Autodesk Inventor part; units mm, degrees
(part 3 of 3)
  spline S382 degree 2 poles (128.7534, 1.3553) (128.7534, 1.4377) (128.7421, 1.5996) (128.7335, 1.6763) knots 0 0 0 1 2 2 2
  line L586 (128.7335, 1.6763) -> (127.3928, 0.6822)
  spline S383 degree 2 poles (127.3928, 0.6822) (127.4269, 0.5543) (127.5405, 0.3413) (127.6968, 0.1879) (127.8984, 0.1027) (128.0291, 0.1027) knots 0 0 0 1 2 3 4 4 4
  spline S384 degree 2 poles (128.0291, 0.1027) (128.1938, 0.1027) (128.4609, 0.2618) (128.6512, 0.5799) (128.7534, 1.0486) (128.7534, 1.3553) knots 0 0 0 1 2 3 4 4 4
  spline S385 degree 2 poles (127.3019, 1.3838) (127.3019, 1.3099) (127.3048, 1.1594) (127.3104, 1.0883) knots 0 0 0 1 2 2 2
  line L587 (127.3104, 1.0883) -> (128.654, 2.0797)
  spline S386 degree 2 poles (128.654, 2.0797) (128.6171, 2.2047) (128.5063, 2.4092) (128.3501, 2.5569) (128.1512, 2.6393) (128.0291, 2.6393) knots 0 0 0 1 2 3 4 4 4
  spline S387 degree 2 poles (128.0291, 2.6393) (127.8615, 2.6393) (127.5945, 2.4802) (127.4042, 2.1621) (127.3019, 1.6934) (127.3019, 1.3838) knots 0 0 0 1 2 3 4 4 4
  line L588 (131.5229, -0.2154) -> (131.5229, 1.5343)
  spline S388 degree 2 poles (131.5229, 1.5343) (131.5229, 1.6479) (131.5059, 1.7928) (131.4718, 1.878) (131.4207, 1.9121) (131.3809, 1.9121) knots 0 0 0 1 2 3 4 4 4
  spline S389 degree 2 poles (131.3809, 1.9121) (131.3354, 1.9121) (131.2587, 1.8553) (131.1707, 1.7218) (131.0656, 1.5059) (130.9917, 1.3497) knots 0 0 0 1 2 3 4 4 4
  line L589 (130.9917, 1.3497) -> (130.9917, -0.2154)
  line L590 (130.9917, -0.2154) -> (130.5685, -0.2154)
  line L591 (130.5685, -0.2154) -> (130.5685, 1.4889)
  spline S390 degree 2 poles (130.5685, 1.4889) (130.5685, 1.6224) (130.5515, 1.7871) (130.5174, 1.878) (130.4634, 1.9121) (130.4236, 1.9121) knots 0 0 0 1 2 3 4 4 4
  spline S391 degree 2 poles (130.4236, 1.9121) (130.3839, 1.9121) (130.31, 1.8638) (130.222, 1.7388) (130.1112, 1.5201) (130.0373, 1.3497) knots 0 0 0 1 2 3 4 4 4
  line L592 (130.0373, 1.3497) -> (130.0373, -0.2154)
  line L593 (130.0373, -0.2154) -> (129.6141, -0.2154)
  line L594 (129.6141, -0.2154) -> (129.6141, 2.2189)
  line L595 (129.6141, 2.2189) -> (129.9663, 2.2189)
  line L596 (129.9663, 2.2189) -> (129.9862, 1.7559)
  spline S392 degree 2 poles (129.9862, 1.7559) (130.0515, 1.895) (130.1708, 2.0882) (130.2958, 2.2075) (130.4407, 2.2643) (130.5259, 2.2643) knots 0 0 0 1 2 3 4 4 4
  spline S393 degree 2 poles (130.5259, 2.2643) (130.7247, 2.2643) (130.9292, 2.0058) (130.9292, 1.736) knots 0 0 0 1 2 2 2
  spline S394 degree 2 poles (130.9292, 1.736) (130.9861, 1.8638) (131.0997, 2.0598) (131.2275, 2.1933) (131.3837, 2.2643) (131.486, 2.2643) knots 0 0 0 1 2 3 4 4 4
  spline S395 degree 2 poles (131.486, 2.2643) (131.9461, 2.2643) (131.9461, 1.557) knots 0 0 0 1 1 1
  line L597 (131.9461, 1.557) -> (131.9461, -0.2154)
  line L598 (131.9461, -0.2154) -> (131.5229, -0.2154)
  line L599 (134.8378, -0.2154) -> (134.3663, -0.2154)
  line L600 (134.3663, -0.2154) -> (134.1475, 0.4748)
  line L601 (134.1475, 0.4748) -> (132.821, 0.4748)
  line L602 (132.821, 0.4748) -> (132.5995, -0.2154)
  line L603 (132.5995, -0.2154) -> (132.1535, -0.2154)
  line L604 (132.1535, -0.2154) -> (133.2045, 2.9546)
  line L605 (133.2045, 2.9546) -> (133.7982, 2.9546)
  line L606 (133.7982, 2.9546) -> (134.8378, -0.2154)
  line L607 (134.0226, 0.8611) -> (133.4857, 2.5597)
  line L608 (133.4857, 2.5597) -> (132.9432, 0.8611)
  line L609 (132.9432, 0.8611) -> (134.0226, 0.8611)
  line L610 (114.9596, -5.248) -> (113.2868, -5.248)
  line L611 (113.2868, -5.248) -> (113.2868, -4.9453)
  line L612 (113.2868, -4.9453) -> (113.9423, -4.2921)
  spline S396 degree 2 poles (113.9423, -4.2921) (114.1039, -4.1328) (114.3064, -3.8984) (114.4179, -3.7049) (114.4566, -3.5342) (114.4566, -3.4363) knots 0 0 0 1 2 3 4 4 4
  spline S397 degree 2 poles (114.4566, -3.4363) (114.4566, -3.343) (114.4066, -3.1746) (114.3019, -3.0449) (114.1334, -2.972) (114.0174, -2.972) knots 0 0 0 1 2 3 4 4 4
  spline S398 degree 2 poles (114.0174, -2.972) (113.8558, -2.972) (113.5918, -3.1154) (113.4825, -3.2315) knots 0 0 0 1 2 2 2
  line L613 (113.4825, -3.2315) -> (113.2959, -3.0062)
  spline S399 degree 2 poles (113.2959, -3.0062) (113.4393, -2.856) (113.8148, -2.6716) (114.0629, -2.6716) knots 0 0 0 1 2 2 2
  spline S400 degree 2 poles (114.0629, -2.6716) (114.2313, -2.6716) (114.5113, -2.7718) (114.7115, -2.9629) (114.8231, -3.2383) (114.8231, -3.4113) knots 0 0 0 1 2 3 4 4 4
  spline S401 degree 2 poles (114.8231, -3.4113) (114.8231, -3.5592) (114.7457, -3.8073) (114.5886, -4.0531) (114.3497, -4.3171) (114.1858, -4.4765) knots 0 0 0 1 2 3 4 4 4
  line L614 (114.1858, -4.4765) -> (113.726, -4.9248)
  line L615 (113.726, -4.9248) -> (114.9596, -4.9248)
  line L616 (114.9596, -4.9248) -> (114.9596, -5.248)
  line L617 (117.2766, -4.6859) -> (116.8419, -4.6859)
  line L618 (116.8419, -4.6859) -> (116.8419, -5.248)
  line L619 (116.8419, -5.248) -> (116.4959, -5.248)
  line L620 (116.4959, -5.248) -> (116.4959, -4.6859)
  line L621 (116.4959, -4.6859) -> (115.2737, -4.6859)
  line L622 (115.2737, -4.6859) -> (115.2737, -4.3877)
  line L623 (115.2737, -4.3877) -> (116.3571, -2.708)
  line L624 (116.3571, -2.708) -> (116.8419, -2.708)
  line L625 (116.8419, -2.708) -> (116.8419, -4.3877)
  line L626 (116.8419, -4.3877) -> (117.2766, -4.3877)
  line L627 (117.2766, -4.3877) -> (117.2766, -4.6859)
  line L628 (116.4959, -3.0335) -> (115.6128, -4.3877)
  line L629 (115.6128, -4.3877) -> (116.4959, -4.3877)
  line L630 (116.4959, -4.3877) -> (116.4959, -3.0335)
  line L631 (117.511, -3.2975) -> (117.8956, -3.2975)
  line L632 (117.8956, -3.2975) -> (118.3713, -4.588)
  line L633 (118.3713, -4.588) -> (118.476, -4.9044)
  line L634 (118.476, -4.9044) -> (118.5807, -4.5812)
  line L635 (118.5807, -4.5812) -> (119.0541, -3.2975)
  line L636 (119.0541, -3.2975) -> (119.4274, -3.2975)
  line L637 (119.4274, -3.2975) -> (118.6604, -5.248)
  line L638 (118.6604, -5.248) -> (118.2735, -5.248)
  line L639 (118.2735, -5.248) -> (117.511, -3.2975)
  spline S402 degree 2 poles (121.6146, -3.9507) (121.6146, -4.1328) (121.5577, -4.4674) (121.4348, -4.7541) (121.2368, -4.9886) (120.9477, -5.157) (120.5677, -5.248) (120.3241, -5.248) knots 0 0 0 1 2 3 4 5 6 6 6
  line L640 (120.3241, -5.248) -> (119.7802, -5.248)
  line L641 (119.7802, -5.248) -> (119.7802, -2.708)
  line L642 (119.7802, -2.708) -> (120.4356, -2.708)
  spline S403 degree 2 poles (120.4356, -2.708) (121.0297, -2.708) (121.6146, -3.3203) (121.6146, -3.9507) knots 0 0 0 1 2 2 2
  spline S404 degree 2 poles (121.2504, -3.9735) (121.2504, -3.7049) (121.1503, -3.3316) (120.9432, -3.1018) (120.6337, -2.9994) (120.4243, -2.9994) knots 0 0 0 1 2 3 4 4 4
  line L643 (120.4243, -2.9994) -> (120.1261, -2.9994)
  line L644 (120.1261, -2.9994) -> (120.1261, -4.9476)
  line L645 (120.1261, -4.9476) -> (120.3833, -4.9476)
  spline S405 degree 2 poles (120.3833, -4.9476) (121.2504, -4.9476) (121.2504, -3.9735) knots 0 0 0 1 1 1
  spline S406 degree 2 poles (123.6926, -5.1524) (123.3876, -5.2799) (123.053, -5.2799) knots 0 0 0 1 1 1
  spline S407 degree 2 poles (123.053, -5.2799) (122.5159, -5.2799) (121.9378, -4.6358) (121.9378, -4.0053) knots 0 0 0 1 2 2 2
  spline S408 degree 2 poles (121.9378, -4.0053) (121.9378, -3.7004) (122.0971, -3.2065) (122.393, -2.8628) (122.8118, -2.6762) (123.0735, -2.6762) knots 0 0 0 1 2 3 4 4 4
  spline S409 degree 2 poles (123.0735, -2.6762) (123.2488, -2.6762) (123.5537, -2.7376) (123.6926, -2.7991) knots 0 0 0 1 2 2 2
  line L646 (123.6926, -2.7991) -> (123.6926, -3.1382)
  spline S410 degree 2 poles (123.6926, -3.1382) (123.5537, -3.0631) (123.2579, -2.9834) (123.0849, -2.9834) knots 0 0 0 1 2 2 2
  spline S411 degree 2 poles (123.0849, -2.9834) (122.9051, -2.9834) (122.616, -3.1177) (122.4135, -3.3726) (122.3042, -3.739) (122.3042, -3.9757) knots 0 0 0 1 2 3 4 4 4
  spline S412 degree 2 poles (122.3042, -3.9757) (122.3042, -4.4696) (122.7048, -4.9704) (123.0917, -4.9704) knots 0 0 0 1 2 2 2
  spline S413 degree 2 poles (123.0917, -4.9704) (123.2556, -4.9704) (123.5537, -4.8952) (123.6926, -4.827) knots 0 0 0 1 2 2 2
  line L647 (123.6926, -4.827) -> (123.6926, -5.1524)
  spline S414 degree 2 poles (127.6141, -6.0651) (126.7196, -5.2344) (126.7196, -4.2284) knots 0 0 0 1 1 1
  spline S415 degree 2 poles (126.7196, -4.2284) (126.7196, -3.994) (126.8152, -3.5251) (127.0269, -3.054) (127.3751, -2.5851) (127.6232, -2.353) knots 0 0 0 1 2 3 4 4 4
  line L648 (127.6232, -2.353) -> (127.8189, -2.5533)
  spline S416 degree 2 poles (127.8189, -2.5533) (127.0656, -3.2975) (127.0656, -4.2033) knots 0 0 0 1 1 1
  spline S417 degree 2 poles (127.0656, -4.2033) (127.0656, -4.6563) (127.4457, -5.487) (127.8189, -5.858) knots 0 0 0 1 2 2 2
  line L649 (127.8189, -5.858) -> (127.6141, -6.0651)
  line L650 (130.4204, -5.248) -> (130.0813, -5.248)
  line L651 (130.0813, -5.248) -> (130.0312, -3.6617)
  line L652 (130.0312, -3.6617) -> (130.0107, -3.0563)
  line L653 (130.0107, -3.0563) -> (129.8924, -3.409)
  line L654 (129.8924, -3.409) -> (129.5168, -4.4196)
  line L655 (129.5168, -4.4196) -> (129.2778, -4.4196)
  line L656 (129.2778, -4.4196) -> (128.9205, -3.4477)
  line L657 (128.9205, -3.4477) -> (128.8044, -3.0563)
  line L658 (128.8044, -3.0563) -> (128.7953, -3.689)
  line L659 (128.7953, -3.689) -> (128.7498, -5.248)
  line L660 (128.7498, -5.248) -> (128.4244, -5.248)
  line L661 (128.4244, -5.248) -> (128.5495, -2.708)
  line L662 (128.5495, -2.708) -> (128.9592, -2.708)
  line L663 (128.9592, -2.708) -> (129.3006, -3.6639)
  line L664 (129.3006, -3.6639) -> (129.4099, -3.9871)
  line L665 (129.4099, -3.9871) -> (129.5168, -3.6639)
  line L666 (129.5168, -3.6639) -> (129.8764, -2.708)
  line L667 (129.8764, -2.708) -> (130.2975, -2.708)
  line L668 (130.2975, -2.708) -> (130.4204, -5.248)
  line L669 (132.0819, -5.248) -> (132.075, -4.9863)
  spline S418 degree 2 poles (132.075, -4.9863) (131.9157, -5.1433) (131.5857, -5.2822) (131.4059, -5.2822) knots 0 0 0 1 2 2 2
  spline S419 degree 2 poles (131.4059, -5.2822) (131.2375, -5.2822) (131.0008, -5.1957) (130.8483, -5.0477) (130.7754, -4.8452) (130.7754, -4.7268) knots 0 0 0 1 2 3 4 4 4
  spline S420 degree 2 poles (130.7754, -4.7268) (130.7754, -4.4332) (131.2124, -4.1009) (131.6403, -4.1009) knots 0 0 0 1 2 2 2
  line L670 (131.6403, -4.1009) -> (132.0454, -4.1009)
  line L671 (132.0454, -4.1009) -> (132.0454, -3.9302)
  spline S421 degree 2 poles (132.0454, -3.9302) (132.0454, -3.7573) (131.8247, -3.5479) (131.5971, -3.5479) knots 0 0 0 1 2 2 2
  spline S422 degree 2 poles (131.5971, -3.5479) (131.4309, -3.5479) (131.11, -3.6207) (130.9393, -3.689) knots 0 0 0 1 2 2 2
  line L672 (130.9393, -3.689) -> (130.9393, -3.384)
  spline S423 degree 2 poles (130.9393, -3.384) (131.003, -3.3612) (131.1601, -3.3157) (131.3353, -3.2816) (131.5265, -3.2611) (131.6221, -3.2611) knots 0 0 0 1 2 3 4 4 4
  spline S424 degree 2 poles (131.6221, -3.2611) (131.7996, -3.2611) (132.0841, -3.3385) (132.2799, -3.4978) (132.3846, -3.739) (132.3846, -3.9029) knots 0 0 0 1 2 3 4 4 4
  line L673 (132.3846, -3.9029) -> (132.3846, -5.248)
  line L674 (132.3846, -5.248) -> (132.0819, -5.248)
  line L675 (132.0454, -4.3604) -> (131.6153, -4.3604)
  spline S425 degree 2 poles (131.6153, -4.3604) (131.4878, -4.3604) (131.3058, -4.4105) (131.1897, -4.5038) (131.1328, -4.6335) (131.1328, -4.7154) knots 0 0 0 1 2 3 4 4 4
  spline S426 degree 2 poles (131.1328, -4.7154) (131.1328, -4.7723) (131.1669, -4.8748) (131.2466, -4.9544) (131.3695, -4.9999) (131.4605, -4.9999) knots 0 0 0 1 2 3 4 4 4
  spline S427 degree 2 poles (131.4605, -4.9999) (131.5766, -4.9999) (131.877, -4.8588) (132.0454, -4.7063) knots 0 0 0 1 2 2 2
  line L676 (132.0454, -4.7063) -> (132.0454, -4.3604)
  line L677 (134.7766, -5.248) -> (134.3283, -5.248)
  line L678 (134.3283, -5.248) -> (133.8002, -4.5061)
  line L679 (133.8002, -4.5061) -> (133.279, -5.248)
  line L680 (133.279, -5.248) -> (132.842, -5.248)
  line L681 (132.842, -5.248) -> (133.5999, -4.2694)
  line L682 (133.5999, -4.2694) -> (132.8762, -3.2975)
  line L683 (132.8762, -3.2975) -> (133.3086, -3.2975)
  line L684 (133.3086, -3.2975) -> (133.823, -4.0486)
  line L685 (133.823, -4.0486) -> (134.326, -3.2975)
  line L686 (134.326, -3.2975) -> (134.7448, -3.2975)
  line L687 (134.7448, -3.2975) -> (134.0119, -4.2762)
  line L688 (134.0119, -4.2762) -> (134.7766, -5.248)
  spline S428 degree 2 poles (135.6051, -2.353) (136.5018, -3.1837) (136.5018, -4.2011) knots 0 0 0 1 1 1
  spline S429 degree 2 poles (136.5018, -4.2011) (136.5018, -4.4105) (136.4153, -4.8611) (136.2105, -5.3345) (135.8623, -5.8193) (135.596, -6.0651) knots 0 0 0 1 2 3 4 4 4
  line L689 (135.596, -6.0651) -> (135.4003, -5.8648)
  spline S430 degree 2 poles (135.4003, -5.8648) (135.7803, -5.4893) (136.1536, -4.6722) (136.1536, -4.2261) knots 0 0 0 1 2 2 2
  spline S431 degree 2 poles (136.1536, -4.2261) (136.1536, -3.2998) (135.4003, -2.5601) knots 0 0 0 1 1 1
  line L690 (135.4003, -2.5601) -> (135.6051, -2.353)
  line L691 (120.7098, -38.17) -> (120.2383, -38.17)
  line L692 (120.2383, -38.17) -> (120.0196, -37.4798)
  line L693 (120.0196, -37.4798) -> (118.6931, -37.4798)
  line L694 (118.6931, -37.4798) -> (118.4715, -38.17)
  line L695 (118.4715, -38.17) -> (118.0256, -38.17)
  line L696 (118.0256, -38.17) -> (119.0766, -35)
  line L697 (119.0766, -35) -> (119.6702, -35)
  line L698 (119.6702, -35) -> (120.7098, -38.17)
  line L699 (119.8946, -37.0934) -> (119.3578, -35.3948)
  line L700 (119.3578, -35.3948) -> (118.8152, -37.0934)
  line L701 (118.8152, -37.0934) -> (119.8946, -37.0934)
  line L702 (121.8801, -35.3636) -> (121.1501, -35.3636)
  line L703 (121.1501, -35.3636) -> (121.1501, -35)
  line L704 (121.1501, -35) -> (123.0476, -35)
  line L705 (123.0476, -35) -> (123.0476, -35.3636)
  line L706 (123.0476, -35.3636) -> (122.3176, -35.3636)
  line L707 (122.3176, -35.3636) -> (122.3176, -37.8007)
  line L708 (122.3176, -37.8007) -> (123.0476, -37.8007)
  line L709 (123.0476, -37.8007) -> (123.0476, -38.17)
  line L710 (123.0476, -38.17) -> (121.1501, -38.17)
  line L711 (121.1501, -38.17) -> (121.1501, -37.8007)
  line L712 (121.1501, -37.8007) -> (121.8801, -37.8007)
  line L713 (121.8801, -37.8007) -> (121.8801, -35.3636)
  line L714 (128.8024, -37.4684) -> (128.2599, -37.4684)
  line L715 (128.2599, -37.4684) -> (128.2599, -38.17)
  line L716 (128.2599, -38.17) -> (127.8281, -38.17)
  line L717 (127.8281, -38.17) -> (127.8281, -37.4684)
  line L718 (127.8281, -37.4684) -> (126.3028, -37.4684)
  line L719 (126.3028, -37.4684) -> (126.3028, -37.0963)
  line L720 (126.3028, -37.0963) -> (127.6549, -35)
  line L721 (127.6549, -35) -> (128.2599, -35)
  line L722 (128.2599, -35) -> (128.2599, -37.0963)
  line L723 (128.2599, -37.0963) -> (128.8024, -37.0963)
  line L724 (128.8024, -37.0963) -> (128.8024, -37.4684)
  line L725 (127.8281, -35.4062) -> (126.726, -37.0963)
  line L726 (126.726, -37.0963) -> (127.8281, -37.0963)
  line L727 (127.8281, -37.0963) -> (127.8281, -35.4062)
  line L728 (75.7098, -38.2154) -> (75.2383, -38.2154)
  line L729 (75.2383, -38.2154) -> (75.0196, -37.5252)
  line L730 (75.0196, -37.5252) -> (73.6931, -37.5252)
  line L731 (73.6931, -37.5252) -> (73.4715, -38.2154)
  line L732 (73.4715, -38.2154) -> (73.0256, -38.2154)
  line L733 (73.0256, -38.2154) -> (74.0766, -35.0454)
  line L734 (74.0766, -35.0454) -> (74.6702, -35.0454)
  line L735 (74.6702, -35.0454) -> (75.7098, -38.2154)
  line L736 (74.8946, -37.1389) -> (74.3578, -35.4403)
  line L737 (74.3578, -35.4403) -> (73.8152, -37.1389)
  line L738 (73.8152, -37.1389) -> (74.8946, -37.1389)
  line L739 (76.8801, -35.409) -> (76.1501, -35.409)
  line L740 (76.1501, -35.409) -> (76.1501, -35.0454)
  line L741 (76.1501, -35.0454) -> (78.0476, -35.0454)
  line L742 (78.0476, -35.0454) -> (78.0476, -35.409)
  line L743 (78.0476, -35.409) -> (77.3176, -35.409)
  line L744 (77.3176, -35.409) -> (77.3176, -37.8462)
  line L745 (77.3176, -37.8462) -> (78.0476, -37.8462)
  line L746 (78.0476, -37.8462) -> (78.0476, -38.2154)
  line L747 (78.0476, -38.2154) -> (76.1501, -38.2154)
  line L748 (76.1501, -38.2154) -> (76.1501, -37.8462)
  line L749 (76.1501, -37.8462) -> (76.8801, -37.8462)
  line L750 (76.8801, -37.8462) -> (76.8801, -35.409)
  line L751 (83.6434, -38.2154) -> (81.5556, -38.2154)
  line L752 (81.5556, -38.2154) -> (81.5556, -37.8377)
  line L753 (81.5556, -37.8377) -> (82.3737, -37.0224)
  spline S432 degree 2 poles (82.3737, -37.0224) (82.5753, -36.8236) (82.8281, -36.531) (82.9673, -36.2896) (83.0156, -36.0766) (83.0156, -35.9544) knots 0 0 0 1 2 3 4 4 4
  spline S433 degree 2 poles (83.0156, -35.9544) (83.0156, -35.8379) (82.9531, -35.6278) (82.8225, -35.4658) (82.6123, -35.3749) (82.4674, -35.3749) knots 0 0 0 1 2 3 4 4 4
  spline S434 degree 2 poles (82.4674, -35.3749) (82.2657, -35.3749) (81.9362, -35.5539) (81.7999, -35.6988) knots 0 0 0 1 2 2 2
  line L754 (81.7999, -35.6988) -> (81.567, -35.4176)
  spline S435 degree 2 poles (81.567, -35.4176) (81.7459, -35.2301) (82.2146, -35) (82.5242, -35) knots 0 0 0 1 2 2 2
  spline S436 degree 2 poles (82.5242, -35) (82.7344, -35) (83.0838, -35.125) (83.3337, -35.3636) (83.4729, -35.7073) (83.4729, -35.9232) knots 0 0 0 1 2 3 4 4 4
  spline S437 degree 2 poles (83.4729, -35.9232) (83.4729, -36.1078) (83.3764, -36.4174) (83.1804, -36.7242) (82.8821, -37.0537) (82.6776, -37.2525) knots 0 0 0 1 2 3 4 4 4
  line L755 (82.6776, -37.2525) -> (82.1038, -37.8121)
  line L756 (82.1038, -37.8121) -> (83.6434, -37.8121)
  line L757 (83.6434, -37.8121) -> (83.6434, -38.2154)
  point P0 (0, 0)
  dimension "d66" = 10
  dimension "d67" = 10
  dimension "d68" = 5
  dimension "d69" = 5
  dimension "d70" = 10
  dimension "d71" = 6
  dimension "d72" = 6
  dimension "d73" = 10
  dimension "d74" = 27
  dimension "d75" = 11
  dimension "d76" = 11
  dimension "d77" = 11
  dimension "d79" = 11
  dimension "d80" = 10
  dimension "d81" = 10
  dimension "d82" = 23
  dimension "d83" = 23
  dimension "d84" = 4
  constraints: 6 horizontal alignment, 4 vertical alignment, 2 horizontal, 28 other
  measures "d66" distance from line of L13 A0.centre
  measures "d67" distance from line of L21 A1.centre
  measures "d68" distance from line of L12 A0.centre
  measures "d69" distance from line of A2.centre L16
  measures "d70" distance from line of L41 A3.centre
  measures "d71" distance from line of A3.centre L40
  measures "d72" distance from line of L48 A4.centre
  measures "d73" distance from line of A5.centre L45
  measures "d74" distance from line of A3.centre L29
  measures "d75" distance from line of A3.centre L28
  measures "d76" distance from line of A4.centre L32
  measures "d77" distance from line of A4.centre L36
  measures "d79" distance between parallel lines of L56 L4
  measures "d80" distance between parallel lines of L57 L7
  measures "d81" distance between parallel lines of L58 L5
  measures "d82" distance from line of A6.centre L8
  measures "d83" distance from line of L10 A6.centre
  measures "d84" distance between parallel lines of L59 L0
extrude "Extrusion4" cut sketch "Sketch5" against normal blind 10 contours L60 L61 L62 L63 L64 L65 | L66 S0 S1 S2 L67 L68 S3 S4 L69 S5 S6 L70 L71 | S10 S11 L74 L75 L76 L77 S12 S13 | L79 L80 L81 L82 L83 L84 L85 L86 L87 | L88 L89 L90 L91 L92 L93 L94 L95 L96 L97 L98 L99 | L100 L101 L102 L103 L104 L105 L106 L107 L108 L109 L110 L111 | L112 L113 L114 L115 L116 L117 L118 L119 L120 L121 L122 L123 L124 L125 L126 L127 L128 L129 L130 | L131 L132 L133 L134 L135 L136 L137 L138 | L139 L140 S18 S19 L141 S20 S21 L142 L143 L144 | L145 S22 S23 S24 L146 L147 S25 S26 L148 S27 S28 L149 L150 | L153 L154 L155 L156 L157 L158 L159 L160 L161 L162 | S32 S33 S34 S35 | L163 L164 S36 S37 L165 L166 L167 S38 S39 L168 L169 L170 | L171 L172 L173 L174 L175 L176 L177 L178 L179 L180 | S40 S41 S42 S43 | L181 L182 S44 S45 L183 L184 L185 S46 S47 L186 L187 L188 | S48 S49 S50 S51 S52 L189 S53 S54 S55 S56 S57 S58 S59 S60 S61 L190 L191 L192 | L194 L195 S70 L196 L197 L198 L199 L200 S71 S72 S73 L201 | L205 L206 L207 L208 L209 L210 L211 L212 L213 L214 | S76 S77 S78 S79 | S80 S81 S82 S83 S84 L215 S85 S86 S87 S88 S89 S90 S91 S92 S93 L216 L217 L218 | L220 L221 L222 L223 L224 L225 L226 L227 | L231 S102 S103 L232 L233 L234 S104 S105 L235 L236 L237 L238 L239 S106 S107 S108 S109 L240 L241 | S110 S111 L242 L243 L244 L245 L246 S112 S113 | L248 S118 S119 L249 L250 L251 S120 S121 L252 L253 L254 L255 L256 S122 S123 S124 S125 L257 L258 | S126 L259 S127 S128 L260 S129 S130 S131 S132 | S135 S136 L262 L263 L264 L265 L266 L267 L268 L269 L270 L271 L272 S137 S138 L273 | S139 L274 S140 S141 L275 S142 S143 S144 S145 | L277 L278 S148 S149 L279 S150 S151 L280 L281 L282 | S152 S153 S154 S155 | L285 L286 L287 L288 | L289 L290 L291 S162 S163 S164 L292 S165 S166 S167 L293 L294 L295 | S168 S169 S170 S171 | L298 S178 S179 L299 L300 L301 S180 S181 L302 L303 L304 L305 L306 S182 S183 S184 S185 L307 L308 | L309 L310 L311 L312 L313 L314 L315 L316 | L320 L321 L322 L323 L324 L325 L326 L327 L328 | S186 S187 S188 S189 | L329 L330 L331 L332 L333 L334 L335 L336 L337 L338 | S194 S195 L339 L340 L341 L342 L343 L344 L345 L346 L347 L348 L349 S196 S197 L350 | L351 S198 S199 L352 L353 L354 S200 S201 L355 L356 L357 L358 L359 S202 S203 S204 S205 L360 L361 | S206 L362 S207 S208 L363 S209 S210 S211 S212 | S215 S216 L365 L366 L367 L368 L369 L370 L371 L372 L373 L374 L375 S217 S218 L376 | S219 L377 S220 S221 L378 S222 S223 S224 S225 | L380 L381 S228 S229 L382 S230 S231 L383 L384 L385 | S232 S233 S234 S235 | L388 L389 L390 L391 | L392 L393 L394 L395 L396 L397 L398 L399 L400 L401 L402 | S242 S243 S244 S245 | L405 L406 L407 L408 L409 L410 L411 L412 L413 | S252 L414 L415 L416 S253 | S256 S257 S258 S259 | S264 S265 L420 S266 S267 S268 L421 L422 L423 S269 S270 S271 L424 S272 S273 S274 S275 | S276 L425 L426 L427 S277 | S280 S281 S282 S283 | L431 L432 L433 L434 L435 L436 L437 L438 L439 L440 L441 | S288 L442 L443 L444 S289 | S292 S293 S294 S295 | L448 L449 L450 S300 S301 S302 L451 S303 S304 S305 L452 L453 L454 | S306 L455 L456 L457 S307 | S310 S311 S312 S313 | L461 L462 L463 L464 L465 L466 L467 L468 L469 L470 L471 | L475 L476 L477 L478 L479 L480 L481 L482 | L486 L487 L488 L489 L490 L491 L492 L493 L494 L495 L496 L497 | L498 L499 L500 L501 L502 L503 L504 L505 L506 L507 L508 | S318 S319 S320 S321 | L511 L512 L513 L514 | L515 L516 L517 L518 L519 L520 L521 L522 L523 L524 L525 | S328 S329 S330 S331 | L528 L529 L530 L531 L532 L533 L534 L535 L536 | S338 L537 L538 L539 S339 | S342 S343 S344 S345 L543 S346 S347 S348 S349 L544 | L545 L546 L547 L548 L549 L550 L551 L552 | L556 L557 L558 L559 L560 L561 L562 L563 L564 L565 L566 L567 | S350 S351 L568 S352 S353 S354 L569 L570 L571 S355 S356 S357 L572 S358 S359 S360 S361 | S362 S363 S364 S365 | L575 L576 L577 L578 | L579 L580 L581 S372 S373 S374 L582 S375 S376 S377 L583 L584 L585 | S378 S379 S380 S381 | L588 S388 S389 L589 L590 L591 S390 S391 L592 L593 L594 L595 L596 S392 S393 S394 S395 L597 L598 | L599 L600 L601 L602 L603 L604 L605 L606 | L610 L611 L612 S396 S397 S398 L613 S399 S400 S401 L614 L615 L616 | L617 L618 L619 L620 L621 L622 L623 L624 L625 L626 L627 | L631 L632 L633 L634 L635 L636 L637 L638 L639 | S402 L640 L641 L642 S403 | S406 S407 S408 S409 L646 S410 S411 S412 S413 L647 | S414 S415 L648 S416 S417 L649 | L650 L651 L652 L653 L654 L655 L656 L657 L658 L659 L660 L661 L662 L663 L664 L665 L666 L667 L668 | L669 S418 S419 S420 L670 L671 S421 S422 L672 S423 S424 L673 L674 | L677 L678 L679 L680 L681 L682 L683 L684 L685 L686 L687 L688 | S428 S429 L689 S430 S431 L690 | L691 L692 L693 L694 L695 L696 L697 L698 | L702 L703 L704 L705 L706 L707 L708 L709 L710 L711 L712 L713 | L714 L715 L716 L717 L718 L719 L720 L721 L722 L723 L724 | L728 L729 L730 L731 L732 L733 L734 L735 | L739 L740 L741 L742 L743 L744 L745 L746 L747 L748 L749 L750 | L751 L752 L753 S432 S433 S434 L754 S435 S436 S437 L755 L756 L757
sketch "Sketch6" plane through (0, 5, 0) normal (0, 1, 0) x (1, 0, 0)
  line L0 (79, 30) -> (79, -25) construction
  line L1 (63, 30) -> (63, -25)
  line L2 (95, -25) -> (95, 30)
  arc A0 (95, 30) -> (63, 30) centre (79, 30) ccw
  arc A1 (63, -25) -> (95, -25) centre (79, -25) ccw
  line L3 (124, 30) -> (124, -25) construction
  line L4 (108, 30) -> (108, -25)
  line L5 (140, -25) -> (140, 30)
  arc A2 (140, 30) -> (108, 30) centre (124, 30) ccw
  arc A3 (108, -25) -> (140, -25) centre (124, -25) ccw
  circle A4 centre (79, 30) radius 4.75 projected
  circle A5 centre (124, 30) radius 4.75 projected
  circle A6 centre (124, -25) radius 4.75 projected
  circle A7 centre (79, -25) radius 4.75 projected
  line L6 (124, -25) -> (124, 30) construction
  line L7 (104.2859, -25) -> (104.2859, -25)
  line L8 (143.7141, -25) -> (143.7141, -25)
  line L9 (97, -25) -> (97, 30)
  arc A8 (61, -25) -> (97, -25) centre (79, -25) ccw
  line L10 (79, 30) -> (79, -25) construction
  line L11 (61, 30) -> (61, -25)
  arc A9 (97, 30) -> (61, 30) centre (79, 30) ccw
  line L12 (124, 30) -> (124, -25) construction
  line L13 (106, 30) -> (106, -25)
  line L14 (142, -25) -> (142, 30)
  arc A10 (142, 30) -> (106, 30) centre (124, 30) ccw
  arc A11 (106, -25) -> (142, -25) centre (124, -25) ccw
  point P0 (0, 0)
  point P1 (79, 2.5)
  point P2 (124, 2.5)
  point P3 (124, 2.5)
  point P4 (1.5875, 1.5875)
  point P5 (79, 2.5)
  point P6 (124, 2.5)
  dimension "d89" = 32
  dimension "d90" = 32
  dimension "d92" = 2
  dimension "d93" = 2
  constraints: 40 end point, 16 point on circle, 16 tangent, 8 centre point, 8 concentric, 5 midpoint, 5 parallel
  measures "d89" distance between parallel lines of L2 L1
  measures "d90" distance between parallel lines of L4 L5
  measures "d92" distance between parallel lines of L9 L2
  measures "d93" distance between parallel lines of L14 L5
extrude "Extrusion5" cut sketch "Sketch6" against normal blind 1
sketch "Sketch2" plane through (0, 0, 0) normal (0, 1, 0) x (1, 0, 0)
  line L0 (-144.7476, -50) -> (134.453, -50)
  point P0 (0, 0)
  point P1 (-130, -50)
  point P2 (130, -50)
  constraints: 2 end point, 2 horizontal alignment
bend part "Bend Part3" radius 5 angle 90 line through (-144.7476, 0, 50) along (1, 0, 0) centre toward (0, -1, 0) moving side (0, 0, 1) both sides no
equation "\"d5\" = 0.5 * d2"
equation "\"d6\" = 0.5 * d0"
equation "\"d23\" = 0.5 * d20"
equation "\"d24\" = 0.5 * d19"
body "Solid1"
